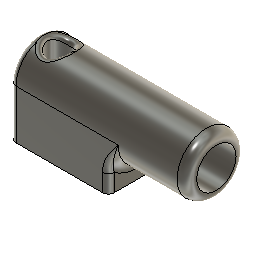
jumpy_door_handle (Autodesk Fusion 360 design; units mm, degrees)
part number: 2026-07-31-21-52-14-922
Autodesk Fusion 360 part; units mm, degrees
sketch "Sketch1" plane through (0, 0, 0) normal (0, 0, 1) x (1, 0, 0)
  line L0 (0, 0) -> (50, 0)
  line L1 (50, 0) -> (50, 30)
  line L2 (50, 30) -> (0, 30)
  line L3 (0, 30) -> (0, 0)
  dimension "d1" = 50
  dimension "d2" = 30
  constraint horizontal L0
  constraint vertical L1
  constraint horizontal L2
  constraint vertical L3
  constraint coincident L0.start L3.end
  measures "d1" distance of L0.start L0.end
  measures "d2" distance of L0.start L2.end
extrude "Extrude1" add sketch "Sketch1" along normal blind 30 makes body 1
sketch "Sketch2" plane through (0, 0, 30) normal (0, 0, 1) x (-1, 0, 0)
  line L0 (0, -30) -> (0, 0)
  line L1 (0, 0) -> (-50, 0)
  line L2 (-50, 0) -> (-50, -30)
  line L3 (-50, -30) -> (0, -30)
  circle A0 centre (-10, -15) radius 3
  line L4 (0, -15) -> (-50, -15) construction
  circle A1 centre (-10, -15) radius 6
  dimension "d5" = 6
  dimension "d6" = 10
  dimension "d9" = 12
  constraint midpoint L0 L4.start
  constraint midpoint L2 L4.end
  constraint coincident A0.centre L4
  constraint concentric A0 A1
  measures "d5" diameter of A0
  measures "d6" distance of L0 A0.centre
  measures "d9" diameter of A1
extrude "Extrude2" cut sketch "Sketch2" against normal blind 40 contours A0 bodies 1
extrude "Extrude3" cut sketch "Sketch2" against normal blind 20 contours A1 bodies 1
sketch "Sketch3" plane through (0, 0, 0) normal (0, 0, -1) x (1, 0, 0)
  circle A0 centre (10, -15) radius 3
  line L0 (0, 0) -> (0, -30)
  line L1 (0, -30) -> (50, -30)
  line L2 (50, -30) -> (50, 0)
  line L3 (50, 0) -> (0, 0)
  line L4 (25, -3) -> (25, -27)
  line L5 (28, 0) -> (28, -30)
  line L6 (25, -3) -> (0, -3)
  line L7 (25, -27) -> (0, -27)
  dimension "d14" = 15
  dimension "d16" = 3
  dimension "d17" = 3
  constraint perpendicular L1 L4
  constraint perpendicular L4 L6
  constraint coincident L0 L7.end
  constraint perpendicular L0 L7
  measures "d14" distance of A0.centre L4
  measures "d16" distance of L3 L6
  measures "d17" distance of L1 L7
extrude "Extrude4" add sketch "Sketch3" along normal blind 10 contours L0 L1 L3 L4 L5 L6 L7 bodies 1
extrude "Extrude5" add 1 faces at (35.3333, 10, 0) along direction (0, 0, -1) blind 10 on bodies 1 bodies 1
sketch "Sketch4" plane through (50, 0, 0) normal (1, 0, 0) x (0, 1, 0)
  line L0 (30, -10) -> (30, 30)
  line L1 (30, 30) -> (0, 30)
  line L2 (0, 30) -> (0, -10)
  line L3 (0, -10) -> (30, -10)
  line L4 (30, 0) -> (0, 0)
  line L5 (0, 0) -> (0, 30)
  line L6 (0, 30) -> (30, 30)
  line L7 (30, 30) -> (30, 0)
  constraint horizontal L4
  constraint vertical L5
  constraint horizontal L6
  constraint vertical L7
  constraint coincident L1.end L2.start
  constraint coincident L0 L4.start
extrude "Extrude6" add sketch "Sketch4" along normal blind 25 contours L0 L1 L2 L4 L5 L6 L7 bodies 1
split "Split1" by plane through (0, 0, 0) normal (0, 0, 1) bodies 1 makes body 2 at (41.6667, 30, 20)
sketch "Sketch5" plane through (0, 0, 0) normal (0, -1, 0) x (1, 0, 0)
  line L0 (0, 0) -> (75, 0)
  line L1 (75, 0) -> (75, 30)
  line L2 (75, 30) -> (0, 30)
  line L3 (0, 30) -> (0, 0)
  line L4 (72, 27) -> (3, 27)
  line L5 (3, 27) -> (3, 3)
  line L6 (3, 3) -> (72, 3)
  line L7 (72, 3) -> (72, 27)
  dimension "d24" = -3
sketch "Sketch6" plane through (0, 30, 0) normal (0, 1, 0) x (-1, 0, 0)
  line L0 (-75, 0) -> (0, 0)
  line L1 (0, 0) -> (0, 30)
  line L2 (0, 30) -> (-75, 30)
  line L3 (-75, 30) -> (-75, 0)
  line L4 (-72, 3) -> (-3, 3)
  line L5 (-3, 3) -> (-3, 27)
  line L6 (-3, 27) -> (-72, 27)
  line L7 (-72, 27) -> (-72, 3)
  dimension "d27" = -3
combine "Combine1" operation add target body 1 tool bodies 2
extrude "Extrude9" add 1 faces at (16.6667, 3, -3.3333) along direction (0, 1, 0) blind 2 on bodies 1 bodies 1
extrude "Extrude10" add 1 faces at (16.6667, 27, -3.3333) along direction (0, -1, 0) blind 2 on bodies 1 bodies 1
sketch "Sketch7" plane through (0, 0, -10) normal (0, 0, -1) x (1, 0, 0)
  line L0 (25, -5) -> (25, -25)
  line L1 (25, -25) -> (0, -25)
  line L2 (0, -25) -> (0, -30)
  line L3 (0, -30) -> (50, -30)
  line L4 (50, -30) -> (50, 0)
  line L5 (50, 0) -> (0, 0)
  line L6 (0, 0) -> (0, -5)
  line L7 (0, -5) -> (25, -5)
  line L8 (27, -5) -> (30, -5)
  line L9 (30, -5) -> (30, -25)
  line L10 (30, -25) -> (27, -25)
  line L11 (27, -25) -> (27, -5)
  dimension "d46" = 2
  dimension "d47" = 3
  constraint horizontal L8
  constraint vertical L9
  constraint horizontal L10
  constraint vertical L11
  measures "d46" distance of L0 L11
  measures "d47" distance of L9 L11
sketch "Sketch8" plane through (75, 0, 0) normal (1, 0, 0) x (0, 1, 0)
  line L0 (30, 30) -> (0, 30)
  line L1 (0, 30) -> (0, 0)
  line L2 (0, 0) -> (30, 0)
  line L3 (30, 0) -> (30, 30)
  circle A0 centre (15, 15) radius 15
  constraint tangent L0 A0
extrude "Extrude12" cut sketch "Sketch8" against normal blind 80 contours L0 L3 A0 | L0 L1 A0 | L2 L3 A0 | L1 L2 A0 bodies 1
extrude "Extrude13" add 2 faces at (41.6667, 6.6667, 0) (41.6667, 23.3333, 0) along direction (0, 0, 1) blind 15 on bodies 1 bodies 1
extrude "Extrude14" add 1 faces at (75, 19.1312, 12.1834) along direction (1, 0, 0) blind 15 on bodies 1 bodies 1
fillet "Fillet9" radius 5 1 faces at (90, 19.1312, 12.1834) on bodies 1
extrude "Extrude15" cut 1 faces at (90, 12.2459, 16.8777) along direction (-1, 0, 0) blind 65 on bodies 1 bodies 1
sketch "Sketch9" plane through (0, 0, -10) normal (0, 0, -1) x (1, 0, 0)
  line L0 (25, -5) -> (25, -25)
  line L1 (25, -25) -> (0, -25)
  line L2 (0, -25) -> (0, -30)
  line L3 (0, -30) -> (50, -30)
  line L4 (50, -30) -> (50, 0)
  line L5 (50, 0) -> (0, 0)
  line L6 (0, 0) -> (0, -5)
  line L7 (0, -5) -> (25, -5)
  line L8 (25, -25) -> (0, -25)
  line L9 (0, -25) -> (0, -5)
  line L10 (0, -5) -> (25, -5)
  line L11 (25, -5) -> (25, -25)
  constraint horizontal L8
  constraint vertical L9
  constraint horizontal L10
  constraint vertical L11
  constraint coincident L6.end L7.start
  constraint coincident L0.end L1.start
extrude "Extrude16" add sketch "Sketch9" against normal blind 14 separate body contours L0 L1 L7 L8 L9 L10 L11 makes body 3
extrude "Extrude17" cut 1 faces at (8.3333, 11.6667, -10) along direction (0, 0, 1) blind 10 on bodies 3 bodies 3
sketch "Sketch10" plane through (0, 0, 4) normal (0, 0, 1) x (-1, 0, 0)
  line L0 (0, -5) -> (-25, -5)
  line L1 (-25, -5) -> (-25, -25)
  line L2 (-25, -25) -> (0, -25)
  line L3 (0, -25) -> (0, -5)
  circle A0 centre (-10, -15) radius 3
  dimension "d66" = 6
  measures "d66" diameter of A0
extrude "Extrude18" cut sketch "Sketch10" against normal blind 8 contours A0 bodies 3
fillet "Fillet10" radius 5 1 edges at (50, 15, 0) on bodies 1
fillet "Fillet11" radius 3 3 edges at (0, 0, 2.5) (0, 15, 30) (0, 30, 2.5) on bodies 1
fillet "Fillet12" radius 3 2 edges at (51.636, 0, 8.6189) (50, 0, -4.1144) on bodies 1
fillet "Fillet13" radius 3 2 edges at (50, 30, -4.1144) (51.636, 30, 8.6189) on bodies 1
combine "Combine2" operation add target body 1 tool bodies 3
sketch "Sketch11" plane through (0, 0, 0) normal (0, 0, -1) x (1, 0, 0)
  line L0 (0, -5) -> (0, -25)
  line L1 (0, -25) -> (25, -25)
  line L2 (25, -25) -> (25, -5)
  line L3 (25, -5) -> (0, -5)
  arc A0 (13, -15) -> (7, -15) centre (10, -15) ccw
  arc A1 (7, -15) -> (13, -15) centre (10, -15) ccw
  line L4 (24, -5) -> (21, -5)
  line L5 (21, -5) -> (21, -25)
  line L6 (21, -25) -> (24, -25)
  line L7 (24, -25) -> (24, -5)
  dimension "d77" = 14
  constraint horizontal L4
  constraint vertical L5
  constraint horizontal L6
  constraint vertical L7
  constraint coincident L1 L5.end
  constraint coincident L3 L4.start
  measures "d77" distance of A0.centre L7
extrude "Extrude19" cut sketch "Sketch11" against normal blind 15 contours L1 L3 L4 L5 L6 L7 bodies 1
extrude "Extrude20" add 1 faces at (25, 11.6667, -6.6667) along direction (-1, 0, 0) blind 1 on bodies 1 bodies 1
fillet "Fillet14" radius 2 1 edges at (21, 15, 0) on bodies 1
fillet "Fillet15" radius 2 2 edges at (10, 9, 28.7477) (10, 21, 28.7477) on bodies 1
fillet "Fillet16" radius 3 1 edges at (25, 11.3838, 5.6767) on bodies 1
